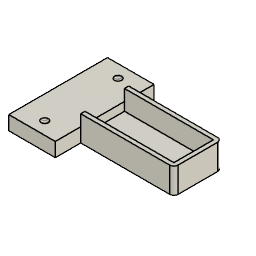
hw-870 sensor holder (Autodesk Fusion 360 design; units mm, degrees)
part number: 2026-03-01-13-27-13-776
Autodesk Fusion 360 part; units mm, degrees
sketch "Schizzo1" plane through (0, 0, 0) normal (0, 0, 1) x (1, 0, 0)
  line L0 (0, 0) -> (31.5, 0)
  line L1 (31.5, 0) -> (31.5, 14)
  line L2 (31.5, 14) -> (0, 14)
  line L3 (0, 14) -> (0, 0)
  line L4 (0, 14) -> (0, 15.5)
  line L5 (0, 15.5) -> (31.5, 15.5)
  line L6 (0, 0) -> (0, -1.5)
  line L7 (0, -1.5) -> (31.5, -1.5)
  line L8 (33, 14) -> (33, 0)
  arc A0 (31.5, -1.5) -> (33, 0) centre (31.5, 0) ccw
  arc A1 (33, 14) -> (31.5, 15.5) centre (31.5, 14) ccw
  line L9 (0, 0) -> (-6.5, 0)
  line L10 (0, 14) -> (-6.5, 14)
  line L11 (-6.5, 14) -> (-6.5, 0)
  line L12 (0, -1.5) -> (-6.5, -1.5)
  line L13 (-6.5, -1.5) -> (-6.5, 0)
  line L14 (-6.5, 14) -> (-6.5, 15.5)
  line L15 (-6.5, 15.5) -> (0, 15.5)
  line L16 (-6.5, 15.5) -> (-16.5, 15.5)
  line L17 (-6.5, 0) -> (-16.5, 0)
  line L18 (-16.5, 15.5) -> (-16.5, 0)
  line L19 (-6.5, -1.5) -> (-16.5, -1.5)
  line L20 (-16.5, -1.5) -> (-16.5, 0)
  line L21 (-6.5, 14) -> (-16.5, 14)
  line L22 (-16.5, -1.5) -> (-16.5, -10.5)
  line L23 (0, -1.5) -> (0, -10.5)
  line L24 (0, -10.5) -> (-16.5, -10.5)
  line L25 (-16.5, 15.5) -> (-16.5, 24.5)
  line L26 (0, 15.5) -> (0, 24.5)
  line L27 (-16.5, 24.5) -> (0, 24.5)
  circle A2 centre (-8.25, -6) radius 1.5
  circle A3 centre (-8.25, 20) radius 1.5
  line L28 (31.5, 0) -> (24.5, 0)
  line L29 (24.5, 1) -> (31, 1)
  line L30 (24.5, 13) -> (31, 13)
  line L31 (31, 13) -> (31, 1)
  line L32 (24.5, 13) -> (24.5, 1)
  dimension "d1" = 31.5
  dimension "d2" = 14
  dimension "d3" = 1.5
  dimension "d4" = 1.5
  dimension "d5" = 1.5
  dimension "d6" = 1.5
  dimension "d7" = 1.5
  dimension "d8" = 1.5
  dimension "d9" = 6.5
  dimension "d10" = 6.5
  dimension "d11" = 10
  dimension "d12" = 10
  dimension "d13" = 9
  dimension "d14" = 9
  dimension "d15" = 9
  dimension "d16" = 9
  dimension "d17" = 3
  dimension "d18" = 3
  dimension "d19" = 7
  dimension "d20" = 1
  dimension "d21" = 6.5
  dimension "d23" = 6.5
  constraint horizontal L0
  constraint vertical L1
  constraint horizontal L2
  constraint vertical L3
  constraint coincident L0.start L3.end
  constraint perpendicular L2 L4
  constraint perpendicular L0 L6
  constraint coincident L0.end L1.start
  constraint coincident L1.end L2.start
  constraint perpendicular L3 L9
  constraint perpendicular L3 L10
  constraint perpendicular L6 L12
  constraint perpendicular L9 L13
  constraint perpendicular L10 L14
  constraint perpendicular L14 L16
  constraint perpendicular L13 L17
  constraint perpendicular L13 L19
  constraint perpendicular L17 L20
  constraint coincident L18 L21.end
  constraint perpendicular L18 L21
  constraint perpendicular L19 L22
  constraint perpendicular L7 L23
  constraint perpendicular L16 L25
  constraint perpendicular L15 L26
  constraint perpendicular L1 L28
  constraint perpendicular L8 L30
  constraint perpendicular L29 L31
  constraint perpendicular L29 L32
  measures "d1" distance of L0.start L0.end
  measures "d2" distance of L0.start L2.end
  measures "d3" distance of L1.end L5.end
  measures "d4" distance of L2.end L4.end
  measures "d5" distance of L0.start L6.end
  measures "d6" distance of L0.end L7.end
  measures "d7" distance of L1.end L8.start
  measures "d8" distance of L0.end L8.end
  measures "d9" distance of L0.start L9.end
  measures "d10" distance of L2.end L10.end
  measures "d11" distance of L14.end L16.end
  measures "d12" distance of L9.end L17.end
  measures "d13" distance of L19.end L22.end
  measures "d14" distance of L6.end L23.end
  measures "d15" distance of L16.end L25.end
  measures "d16" distance of L4.end L26.end
  measures "d17" diameter of A2
  measures "d18" diameter of A3
  measures "d19" distance of L0.end L28.end
  measures "d20" distance of L28.end L29.start
  measures "d21" distance of L29.start L29.end
  measures "d23" distance of L30.start L30.end
extrude "Estrusione1" add sketch "Schizzo1" along normal blind 2 contours L0 L1 L2 L3 L28 makes body 1
extrude "Estrusione2" add sketch "Schizzo1" along normal blind 9 contours L0 L1 L2 L4 L5 L6 L7 L8 A0 A1 L28 bodies 1
extrude "Estrusione3" add sketch "Schizzo1" along normal blind 5 separate body contours L3 L9 L10 L11 makes body 2
extrude "Estrusione4" add sketch "Schizzo1" along normal blind 5 contours L6 L9 L12 L13 | L4 L10 L14 L15 | L12 L19 L22 L23 L24 | L11 L17 L18 L21 | L13 L17 L19 L20 | L15 L16 L25 L26 L27 | L14 L16 L18 L21 bodies 1 2
extrude "Estrusione5" add sketch "Schizzo1" along normal blind 5 contours A3 bodies 1
extrude "Estrusione6" add sketch "Schizzo1" along normal blind 5 contours A2 bodies 1
hole "Foratura1" at (-8.25, 20, 5) direction (0, 0, -1) diameter 2.529 depth 6 tip angle 118 bodies 1
thread "Filettatura1" "ISO Metric profile 3.0 M3x0.5 M3x0.5 6H" thread offset 0 thread depth 7.4
hole "Foratura2" at (-8.25, -6.0001, 5) direction (0, 0, -1) diameter 2.529 depth 6 tip angle 118 bodies 1
thread "Filettatura2" "ISO Metric profile 3.0 M3x0.5 M3x0.5 6H" thread offset 0 thread depth 7.4
